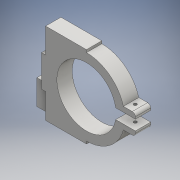
# Autodesk Inventor part: Clamp
Saved by Autodesk Inventor 2016 (Build 200138000, 138)
## iProperties
Created: 2016-04-17
Part Number: Clamp
Material: PC/ABS Plastic
Document SubType Name: Modeling
Designer: amenoni
Density: 0.357273 g/cm^3
Appearance: Smooth - White
Author: amenoni
Autodesk Inventor part; units mm, degrees
ref_plane "YZ Plane" through (0, 0, 0) normal (1, 0, 0) x (0, 1, 0)
ref_plane "XZ Plane" through (0, 0, 0) normal (0, 1, 0) x (-1, 0, 0)
ref_plane "XY Plane" through (0, 0, 0) normal (0, 0, 1) x (1, 0, 0)
sketch "Sketch1" plane through (0, 0, 0) normal (0, 1, 0) x (-1, 0, 0)
  line L0 (-40, -40) -> (40, -40)
  line L1 (40, -40) -> (40, 40)
  line L2 (40, 40) -> (-40, 40)
  line L3 (-40, 40) -> (-40, -40)
  line L4 (-40, -40) -> (40, 40) construction
  line L5 (40, -40) -> (-40, 40) construction
  point P0 (0, 0)
  dimension "d0" = 80
  dimension "d1" = 80
  constraints: 12 end point, 2 midpoint, 2 parallel, 1 horizontal, 1 perpendicular
  measures "d0" distance of L2.end L1.end
  measures "d1" distance of L1.end L0.end
extrude "Extrusion1" add sketch "Sketch1" along normal blind 15
sketch "Sketch2" plane through (0, 15, 0) normal (0, 1, 0) x (1, 0, 0)
  point P0 (0, 0)
  point P1 (0, 0)
  constraints: 1 coincident
hole "Hole1" at (0, 15, 0) direction (0, -1, 0) diameter 58 end through all
sketch "Sketch3" plane through (0, 15, 0) normal (0, 1, 0) x (1, 0, 0)
  arc A0 (0, -37.5) -> (0, 37.5) centre (0, 0) ccw
  line L0 (-40, -40) -> (40, -40) projected
  line L1 (40, -40) -> (40, 40) projected
  line L2 (0, -40) -> (40, -40)
  line L3 (40, -40) -> (40, 40)
  line L4 (40, 40) -> (0, 40)
  line L5 (0, 40) -> (0, 37.5)
  line L6 (0, -37.5) -> (0, -40)
  dimension "d11" = 75
  constraints: 10 end point, 3 parallel, 2 point on circle, 1 centre point, 1 coincident, 1 horizontal, 1 midpoint, 1 perpendicular
  measures "d11" diameter of A0
extrude "Extrusion2" cut sketch "Sketch3" against normal through all
sketch "Sketch4" plane through (0, 15, 0) normal (0, 1, 0) x (1, 0, 0)
  line L0 (41.8017, 5) -> (26.6036, 5)
  line L1 (26.6036, 5) -> (26.6036, -5)
  line L2 (26.6036, -5) -> (41.8017, -5)
  line L3 (41.8017, -5) -> (41.8017, 5)
  line L4 (41.8017, 5) -> (26.6036, -5) construction
  line L5 (26.6036, 5) -> (41.8017, -5) construction
  point P0 (0, 0)
  point P1 (34.2027, 0)
  dimension "d14" = 10
  constraints: 12 end point, 2 midpoint, 2 parallel, 1 horizontal, 1 perpendicular
  measures "d14" distance of L1.end L0.end
extrude "Extrusion3" cut sketch "Sketch4" against normal through all
sketch "Sketch5" plane through (0, 15, 0) normal (0, 1, 0) x (1, 0, 0)
  line L0 (28.5657, -5) -> (37.1652, -5) projected
  line L1 (32.8654, -5) -> (47.8654, -5)
  line L2 (47.8654, -5) -> (47.8654, -10)
  line L3 (47.8654, -10) -> (32.8654, -10)
  line L4 (32.8654, -10) -> (32.8654, -5)
  line L5 (25.4496, 0) -> (55.494, 0)
  line L6 (28.5657, 5) -> (37.1652, 5)
  line L7 (32.8654, 5) -> (47.8654, 5)
  line L8 (47.8654, 5) -> (47.8654, 10)
  line L9 (47.8654, 10) -> (32.8654, 10)
  line L10 (32.8654, 10) -> (32.8654, 5)
  point P0 (0, 0)
  dimension "d17" = 15
  dimension "d18" = 5
  constraints: 20 end point, 6 symmetric about line, 2 horizontal, 2 parallel, 1 midpoint, 1 perpendicular
  measures "d17" distance of L2.end L3.end
  measures "d18" distance of L1.end L2.end
extrude "Extrusion4" add sketch "Sketch5" against normal blind 15
fillet "Fillet1" radius 3 2 edges at (47.8654, 7.5, 10) (47.8654, 7.5, -10)
sketch "Sketch6" plane through (36.1421, 0, 10) normal (0, 0, 1) x (1, 0, 0)
  line L0 (8.7234, 15) -> (8.7234, 0) projected
  point P0 (-36.1421, 0)
  point P1 (4.1079, 7.5)
  dimension "d22" = 4.6155
  measures "d22" distance from line of point (4.108, 7.5) L0
hole "Hole2" at (40.2499, 7.5, 10) direction (0, 0, -1) diameter 3 end through all
sketch "Sketch7" plane through (-40, 0, -40) normal (-1, 0, 0) x (0, 0, 1)
  line L0 (30, 15) -> (2.5, 15) projected
  line L1 (0, 0) -> (80, 0) projected
  line L2 (24.5, 15) -> (55.5, 15)
  line L3 (55.5, 15) -> (55.5, 0)
  line L4 (55.5, 0) -> (24.5, 0)
  line L5 (24.5, 0) -> (24.5, 15)
  line L6 (0, 0) -> (0, 15) projected
  point P0 (40, 0)
  dimension "d30" = 31
  dimension "d31" = 24.5
  constraints: 8 end point, 2 parallel, 2 point on line, 1 horizontal, 1 perpendicular
  measures "d30" distance of L3.end L4.end
  measures "d31" distance between parallel lines of L6 L5
extrude "Extrusion5" add sketch "Sketch7" along normal blind 4
sketch "Sketch8" plane through (-40, 0, -40) normal (-1, 0, 0) x (0, 0, 1)
  line L0 (0, 15) -> (0, 0) projected
  line L1 (24.5, 15) -> (24.5, 0) projected
  line L2 (0, 15) -> (24.5, 15)
  line L3 (24.5, 15) -> (24.5, 7.5)
  line L4 (24.5, 7.5) -> (0, 7.5)
  line L5 (0, 7.5) -> (0, 15)
  point P0 (40, 0)
  dimension "d34" = 7.5
  constraints: 8 end point, 2 parallel, 1 horizontal, 1 midpoint, 1 perpendicular
  measures "d34" distance of L2.end L3.end
extrude "Extrusion6" add sketch "Sketch8" along normal blind 16
body "Solid1"
